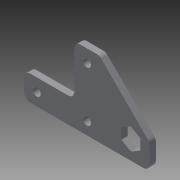
# Autodesk Inventor part: Spacer 3(Left)
Saved by Autodesk Inventor 2014 (Build 180170000, 170)
## iProperties
Created: 2014-01-17
Part Number: Spacer 3(Left)
Material: Generic
Document SubType Name: Sheet Metal
Designer: Michael
Density: 1 g/cm^3
Sheet Metal Rule: Default
Appearance: Default
Author: Michael
Autodesk Inventor part; units mm, degrees
ref_plane "YZ Plane" through (0, 0, 0) normal (1, 0, 0) x (0, 1, 0)
ref_plane "XZ Plane" through (0, 0, 0) normal (0, 1, 0) x (-1, 0, 0)
ref_plane "XY Plane" through (0, 0, 0) normal (0, 0, 1) x (1, 0, 0)
sketch "Sketch1" plane through (0, 0, 0) normal (0, 0, 1) x (1, 0, 0)
  line L0 (0, 0) -> (0, 12.7)
  line L1 (0, 12.7) -> (25.4, 12.7)
  line L2 (25.4, 12.7) -> (25.4, 38.1)
  line L3 (25.4, 38.1) -> (38.1, 38.1)
  line L4 (38.1, 38.1) -> (63.5, 12.7)
  line L5 (63.5, 12.7) -> (63.5, 0)
  line L6 (63.5, 0) -> (0, 0)
  line L7 (49.2125, 12.2746) -> (53.975, 15.0243)
  line L8 (53.975, 15.0243) -> (58.7375, 12.2746)
  line L9 (58.7375, 12.2746) -> (58.7375, 6.7754)
  line L10 (58.7375, 6.7754) -> (53.975, 4.0257)
  line L11 (53.975, 4.0257) -> (49.2125, 6.7754)
  line L12 (49.2125, 6.7754) -> (49.2125, 12.2746)
  circle A0 centre (6.35, 6.35) radius 2.0701
  circle A1 centre (31.75, 6.35) radius 2.0701
  circle A2 centre (31.75, 31.75) radius 2.0701
  point P0 (53.975, 9.525)
  dimension "d0" = 12.7
  dimension "d1" = 25.4
  dimension "d2" = 25.4
  dimension "d3" = 12.7
  dimension "d4" = 63.5
  dimension "d5" = 9.525
  dimension "d6" = 9.525
  dimension "d7" = 9.525
  dimension "d8" = 90
  dimension "d9" = 12.7
  dimension "d10" = 4.1402
  dimension "d11" = 6.35
  dimension "d12" = 6.35
  dimension "d15" = 25.4
  dimension "d22" = 25.4
  measures "d0" distance of L0.start L0.end
  measures "d1" distance of L0.end L1.end
  measures "d2" distance of L1.end L2.end
  measures "d3" distance of L2.end L3.end
  measures "d4" distance of L5.end L0.start
  measures "d5" distance between parallel lines of L12 L9
  measures "d6" distance from line of L6 point (53.975, 9.525)
  measures "d7" distance from line of L5 point (53.975, 9.525)
  measures "d8" angle of L6 L9
  measures "d9" distance of L4.end L5.end
  measures "d10" diameter of A0
  measures "d11" distance from line of L0 A0.centre
  measures "d12" distance from line of L1 A0.centre
  measures "d15" distance of A0.centre A1.centre
  measures "d22" distance of A1.centre A2.centre
extrude "Plate1" add sketch "Sketch1" along normal blind 3.175
fillet "Fillet1" radius 3.175 7 edges at (25.4, 12.7, 1.5875) (0, 12.7, 1.5875) (0, 0, 1.5875) (25.4, 38.1, 1.5875) (38.1, 38.1, 1.5875) (63.5, 12.7, 1.5875) (63.5, 0, 1.5875)
equation "\"BendRadius\" = Thickness"
equation "\"BendReliefWidth\" = Thickness"
equation "\"BendReliefDepth\" = 0.5 * Thickness"
equation "\"CornerReliefSize\" = 4 * Thickness"
equation "\"MinimumRemnant\" = 2 * Thickness"
equation "\"TransitionRadius\" = BendRadius"
equation "\"JacobiRadiusSize\" = BendRadius"
equation "\"GapSize\" = Thickness"
equation "\"d27\" = BendRadius"
equation "\"Thickness\" = 3.175"
body "Solid1"
